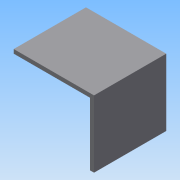
# Autodesk Inventor part: крепление концевика
Saved by Autodesk Inventor 2017 (Build 210142000, 142)
## iProperties
Part Number: крепление концевика
Material: Типовые
Document SubType Name: Modeling
Designer: Max
Mass: 1.87279 g
Surface Area: 28.6859 cm^2
Volume: 1.87279 cm^3
Density: 1 g/cm^3
Appearance: Оружейный металл
Author: Max
Autodesk Inventor part; units mm, degrees
ref_plane "YZ Plane" through (0, 0, 0) normal (1, 0, 0) x (0, 1, 0)
ref_plane "XZ Plane" through (0, 0, 0) normal (0, 1, 0) x (-1, 0, 0)
ref_plane "XY Plane" through (0, 0, 0) normal (0, 0, 1) x (1, 0, 0)
sketch "Эскиз1" plane through (0, 0, 0) normal (0, 1, 0) x (-1, 0, 0)
  line L0 (0, 0) -> (30, 0)
  line L1 (30, 0) -> (30, -1.5)
  line L2 (30, -1.5) -> (0, -1.5)
  line L3 (0, -1.5) -> (0, 0)
  line L4 (0, -1.5) -> (1.5, -1.5)
  line L5 (1.5, -1.5) -> (1.5, -25)
  line L6 (1.5, -25) -> (0, -25)
  line L7 (0, -25) -> (0, -1.5)
  dimension "d0" = 1.5
  dimension "d1" = 25
  dimension "d2" = 30
  dimension "d3" = 1.5
  constraints: 16 end point, 4 parallel, 2 horizontal, 2 perpendicular
  measures "d0" distance between parallel lines of L7 L5
  measures "d1" distance between parallel lines of L0 L6
  measures "d2" distance between parallel lines of L7 L1
  measures "d3" distance between parallel lines of L0 L2
extrude "Выдавливание1" add sketch "Эскиз1" along normal mid plane 27
sketch "Эскиз2" plane through (-1.5, -13.5, -1.5) normal (0, 0, -1) x (-1, 0, 0)
  line L0 (28.5, 27) -> (-1.5, 27) construction
  line L1 (23.581, 27) -> (23.581, 0.3508) construction
  line L2 (28.5, 0) -> (28.5, 27) construction
  line L3 (28.5, 13.5) -> (-1.5, 13.5) construction
  circle A0 centre (23.581, 21) radius 1.5
  circle A1 centre (23.581, 6) radius 1.5
  line L4 (0, 0) -> (0, 27) projected
  line L5 (0, 17.5) -> (15.5309, 17.5)
  line L6 (15.5309, 17.5) -> (15.5309, 9.5)
  line L7 (15.5309, 9.5) -> (0, 9.5)
  line L8 (0, 9.5) -> (0, 17.5)
  line L9 (28.5, 0) -> (0, 0) projected
  dimension "d6" = 3
  dimension "d7" = 3
  dimension "d8" = 15
  dimension "d9" = 7.5
  dimension "d10" = 9.5
  dimension "d11" = 15.5309
  dimension "d12" = 9.5
  constraints: 12 end point, 4 point on line, 2 centre point, 2 horizontal, 2 parallel, 1 midpoint, 1 perpendicular, 1 vertical
  measures "d6" diameter of A0
  measures "d7" diameter of A1
  measures "d8" distance of A1.centre A0.centre
  measures "d9" distance from line of A0.centre L3
  measures "d10" distance between parallel lines of L0 L5
  measures "d11" distance of L6.end L7.end
  measures "d12" distance between parallel lines of L9 L7
extrude "Выдавливание2" cut sketch "Эскиз2" against normal blind 27 contours L4 L5 L6 L7
fillet "Сопряжение1" radius 1 2 edges at (-1.5, 8.75, -1.5) (-1.5, -8.75, -1.5)
fillet "Сопряжение2" radius 3 1 edges at (0, 0, 0)
extrude "Выдавливание3" cut sketch "Эскиз2" against normal blind 27 contours A0 | A1
sketch "Эскиз3" plane through (-1.5, -13.5, -25) normal (-1, 0, 0) x (0, 0, 1)
  circle A0 centre (3.2567, 9.1412) radius 1.5
  circle A1 centre (11.2567, 23.1412) radius 1.5
  point P0 (25, 13.5)
  dimension "d19" = 3
  dimension "d20" = 3
  dimension "d23" = 14
  dimension "d24" = 8
  constraints: 2 centre point
  measures "d19" diameter of A0
  measures "d20" diameter of A1
  measures "d23" vertical distance of A0.centre A1.centre
  measures "d24" horizontal distance of A1.centre A0.centre
extrude "Выдавливание4" cut sketch "Эскиз3" against normal blind 27
fillet "Сопряжение3" radius 5 2 edges at (-30, -13.5, -0.75) (-30, 13.5, -0.75)
fillet "Сопряжение4" radius 2 2 edges at (-0.75, -13.5, -25) (-0.75, 13.5, -25)
